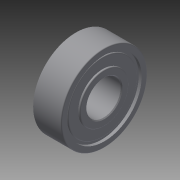
# Autodesk Inventor part: Lozisko_15mm
Saved by Autodesk Inventor 2015 (Build 190159000, 159)
## iProperties
Created: 2015-01-01
Part Number: Lozisko_15mm
Material: Generic
Document SubType Name: Modeling
Designer: Turboslimak
Density: 1 g/cm^3
Appearance: Default
Author: Turboslimak
Autodesk Inventor part; units mm, degrees
ref_plane "YZ Plane" through (0, 0, 0) normal (1, 0, 0) x (0, 1, 0)
ref_plane "XZ Plane" through (0, 0, 0) normal (0, 1, 0) x (-1, 0, 0)
ref_plane "XY Plane" through (0, 0, 0) normal (0, 0, 1) x (1, 0, 0)
sketch "Sketch1" plane through (0, 0, 0) normal (0, 1, 0) x (-1, 0, 0)
  line L0 (-2.5, -4.25) -> (-2.2, -4.25)
  line L1 (-2.2, -4.25) -> (-2.2, -6.05)
  line L2 (-2.2, -6.05) -> (-2, -6.05)
  line L3 (-2.5, -7.5) -> (-2.5, -6.5)
  line L4 (-2.5, -6.5) -> (-2, -6.5)
  line L5 (-2, -6.5) -> (-2, -6.05)
  line L6 (-2.5, 0) -> (0, 0)
  line L7 (0, -7.5) -> (-2.5, -7.5)
  line L8 (2.5, -4.25) -> (2.2, -4.25)
  line L9 (2.2, -4.25) -> (2.2, -6.05)
  line L10 (2.2, -6.05) -> (2, -6.05)
  line L11 (2.5, -6.5) -> (2, -6.5)
  line L12 (2, -6.5) -> (2, -6.05)
  line L13 (2.5, 0) -> (0, 0)
  line L14 (0, -7.5) -> (2.5, -7.5)
  line L15 (2.5, 0) -> (2.5, -4.25)
  line L16 (2.5, -6.5) -> (2.5, -7.5)
  line L17 (-2.5, 0) -> (-2.5, -4.25)
  line L18 (2.5, 0) -> (-2.5, 0)
  line L19 (-2.5, 0) -> (-2.5, -4.25)
  line L20 (-2.5, -4.25) -> (-2.2, -4.25)
  line L21 (-2.2, -6.05) -> (-2, -6.05)
  line L22 (-2, -6.5) -> (-2, -6.05)
  line L23 (-2, -6.5) -> (-2.5, -6.5)
  line L24 (-2.5, -6.5) -> (-2.5, -7.5)
  line L25 (-2.5, -7.5) -> (2.5, -7.5)
  dimension "d2" = 4.25
  dimension "d3" = 0.3
  dimension "d4" = 1.8
  dimension "d5" = 0.2
  dimension "d6" = 1
  dimension "d8" = 2.5
  dimension "d9" = 7.5
  constraints: 52 end point, 5 collinear, 4 perpendicular, 4 vertical, 2 parallel, 1 horizontal
  measures "d2" distance of L6.start L0.start
  measures "d3" distance of L0.start L0.end
  measures "d4" distance of L0.end L1.end
  measures "d5" distance of L1.end L2.end
  measures "d6" distance of L3.start L3.end
  measures "d8" distance of L7.start L7.end
  measures "d9" distance of L6.end L7.start
revolve "Revolution1" add sketch "Sketch1" angle 360 about axis through (-2.5, 0, 0) along (1, 0, 0)
sketch "Sketch2" plane through (-2.5, 0, 0) normal (-1, 0, 0) x (0, 0, 1)
  circle A0 centre (0, 0) radius 3
  dimension "d11" = 6
  constraints: 1 centre point, 1 coincident
  measures "d11" diameter of A0
extrude "Extrusion1" cut sketch "Sketch2" against normal blind 5
chamfer "Chamfer1" distance 0.15 angle 45 1 edges at (-2.5, 0, -3)
chamfer "Chamfer2" distance 0.15 angle 45 1 edges at (2.5, 0, -3)
fillet "Fillet1" radius 0.15 1 edges at (2.5, 0, 4.25)
fillet "Fillet2" radius 0.15 1 edges at (2.2, 0, 6.05)
fillet "Fillet3" radius 0.15 4 edges at (2.5, 0, 7.5) (-2.5, 0, 7.5) (-2.5, 0, 4.25) (-2.2, 0, 6.05)
body "Solid1"
